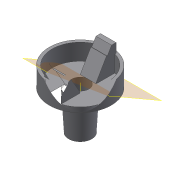
# Autodesk Inventor part: ECoG_holder_2p1
Saved by Autodesk Inventor 2014 (Build 180170000, 170)
## iProperties
Created: 2016-08-28
Part Number: ECoG_holder_2p1
Material: Generic
Document SubType Name: Modeling
Designer: Camilo
Density: 1 g/cm^3
Appearance: Default
Author: Camilo
Autodesk Inventor part; units mm, degrees
ref_plane "YZ Plane" through (0, 0, 0) normal (1, 0, 0) x (0, 1, 0)
ref_plane "XZ Plane" through (0, 0, 0) normal (0, 1, 0) x (-1, 0, 0)
ref_plane "XY Plane" through (0, 0, 0) normal (0, 0, 1) x (1, 0, 0)
sketch "Sketch1" plane through (0, 0, 0) normal (0, 0, 1) x (1, 0, 0)
  circle A0 centre (0, 0) radius 6.94 construction
  circle A1 centre (0, 0) radius 6.93
  point P0 (0, 0)
  dimension "d0" = 0.01
  constraints: 1 centre point, 1 coincident
  measures "d0" radial gap between concentric circles of A0 A1
sketch "Sketch1 outline for Extrusion1" plane through (0, 0, 0) normal (0, 0, 1) x (1, 0, 0)
  circle A0 centre (0, 0) radius 6.93
extrude "Extrusion1" add sketch "Sketch1 outline for Extrusion1" against normal blind 20
sketch "Sketch2" plane through (0, 0, 0) normal (1, 0, 0) x (0, 1, 0)
  line L0 (-6.93, -20) -> (6.93, -20) construction
  line L1 (-6.93, 0) -> (6.93, 0) construction
  line L2 (6.93, -20) -> (6.93, -1.5)
  line L3 (6.93, -1.5) -> (5.93, -20)
  line L4 (6.93, -20) -> (5.93, -20)
  line L5 (0, 4) -> (0, -24) projected
  point P0 (0, 0)
  dimension "d3" = 1.5
  dimension "d4" = 1
  constraints: 6 end point, 1 point on line
  measures "d3" distance from line of L2.end L1
  measures "d4" distance of L0.end L3.end
sketch "Sketch2 outline for Revolution1" plane through (0, 0, 0) normal (1, 0, 0) x (0, 1, 0)
  line L0 (5.93, -20) -> (6.93, -20)
  line L1 (6.93, -1.5) -> (5.93, -20)
  line L2 (6.93, -20) -> (6.93, -1.5)
revolve "Revolution1" cut sketch "Sketch2 outline for Revolution1" angle 360 about axis through (0, 0, 0) along (0, 0, -1)
sketch "Sketch3" plane through (0, 0, 0) normal (0, 0, 1) x (1, 0, 0)
  circle A0 centre (0, 0) radius 6.93 construction
  circle A1 centre (0, 0) radius 14.43
  dimension "d6" = 7.5
  constraints: 1 centre point, 1 coincident
  measures "d6" radial gap between concentric circles of A0 A1
sketch "Sketch3 outline for Extrusion2" plane through (0, 0, 0) normal (0, 0, 1) x (1, 0, 0)
  circle A0 centre (0, 0) radius 14.43
extrude "Extrusion2" add sketch "Sketch3 outline for Extrusion2" along normal blind 1.5
sketch "Sketch4" plane through (0, 0, -20) normal (0, 0, -1) x (-1, 0, 0)
  circle A0 centre (0, 0) radius 5.93 construction
  circle A1 centre (0, 0) radius 4.43
  dimension "d9" = 1.5
  constraints: 1 centre point, 1 coincident
  measures "d9" radial gap between concentric circles of A0 A1
sketch "Sketch4 outline for Extrusion3" plane through (0, 0, -20) normal (0, 0, -1) x (-1, 0, 0)
  circle A0 centre (0, 0) radius 4.43
extrude "Extrusion3" cut sketch "Sketch4 outline for Extrusion3" against normal through all
sketch "Sketch5" plane through (0, 0, 0) normal (1, 0, 0) x (0, 1, 0)
  line L0 (-4.43, 1.5) -> (4.43, 1.5) construction
  line L1 (14.43, 1.5) -> (-14.43, 1.5) construction
  line L2 (4.43, 1.5) -> (14.43, 1.5)
  line L3 (14.43, 1.5) -> (14.43, 18.820508)
  line L4 (14.43, 18.820508) -> (4.43, 1.5)
  point P0 (0, 0)
  dimension "d15" = 60
  constraints: 6 end point, 1 vertical
  measures "d15" angle of L4 L1
sketch "Sketch5 outline for Extrusion4" plane through (0, 0, 0) normal (1, 0, 0) x (0, 1, 0)
  line L0 (14.43, 18.820508) -> (4.43, 1.5)
  line L1 (14.43, 1.5) -> (14.43, 18.820508)
  line L2 (4.43, 1.5) -> (14.43, 1.5)
extrude "Extrusion4" add sketch "Sketch5 outline for Extrusion4" along normal mid plane 8
ref_plane "Work Plane1" through (0, 4.43, 1.5) normal (0, 0.5, 0.8660254) x (-1, 0, 0)
sketch "Sketch6" plane through (-4, 14.43, 18.820508) normal (0, -0.8660254, 0.5) x (1, 0, 0)
  line L0 (0, -20) -> (0, 0)
  line L1 (0.50115, -8.72775) -> (7.50139, -8.72775)
  line L2 (8, -20) -> (0, -20)
  line L3 (0, -20) -> (0, -8.97775)
  line L4 (0, -8.97775) -> (8, -8.97775)
  line L5 (8, -8.97775) -> (8, -20)
  point P0 (4, -23.514038)
  dimension "d16" = 0.25
  constraints: 8 end point, 1 point on line
  measures "d16" distance between parallel lines of L4 L1
sketch "Sketch6 outline for Extrusion5" plane through (-4, 14.43, 18.820508) normal (0, -0.8660254, 0.5) x (1, 0, 0)
  line L0 (0, -20) -> (8, -20)
  line L1 (0, -8.97775) -> (0, -20)
  line L2 (8, -8.97775) -> (0, -8.97775)
  line L3 (8, -20) -> (8, -8.97775)
extrude "Extrusion5" add sketch "Sketch6 outline for Extrusion5" along normal blind 0.5
sketch "Sketch7" plane through (4, 0, 0) normal (1, 0, 0) x (0, 0, -1)
  line L0 (-1.5, 14.43) -> (-18.820508, 14.43) construction
  line L1 (-18.820508, 14.43) -> (-11.045549, 9.941125) construction
  line L2 (-18.820508, 14.43) -> (-14.820508, 14.43)
  line L3 (-18.820508, 14.43) -> (-14.820508, 12.120599)
  line L4 (-14.820508, 14.43) -> (-14.820508, 12.120599)
  point P0 (0, 0)
  dimension "d19" = 4
  constraints: 6 end point, 2 point on line, 1 vertical
  measures "d19" distance of L0.end L2.end
sketch "Sketch7 outline for Extrusion6" plane through (4, 0, 0) normal (1, 0, 0) x (0, 0, -1)
  line L0 (-18.820508, 14.43) -> (-14.820508, 14.43)
  line L1 (-14.820508, 14.43) -> (-14.820508, 12.120599)
  line L2 (-14.820508, 12.120599) -> (-18.820508, 14.43)
extrude "Extrusion6" cut sketch "Sketch7 outline for Extrusion6" against normal up to surface (8 mm away)
sketch "Sketch8" plane through (0, 0, 0) normal (0, 0, -1) x (-1, 0, 0)
  circle A0 centre (0, 0) radius 14.43 construction
  circle A1 centre (0, 0) radius 6.93 construction
  circle A2 centre (0, 0) radius 14.43
  circle A3 centre (0, 0) radius 15.93
  dimension "d22" = 0
  dimension "d23" = 1.5
  constraints: 2 centre point, 2 coincident
  measures "d22" radial gap between concentric circles of A2 A0
  measures "d23" radial gap between concentric circles of A3 A0
sketch "Sketch8 outline for Extrusion7" plane through (0, 0, 0) normal (0, 0, -1) x (-1, 0, 0)
  circle A0 centre (0, 0) radius 15.93
  circle A1 centre (0, 0) radius 14.43
extrude "Extrusion7" add sketch "Sketch8 outline for Extrusion7" against normal blind 10
mirror "Mirror1" about plane through (0, 0, 0) normal (0, 1, 0) of "Extrusion4", "Extrusion5", "Extrusion6"
body "Solid1"
